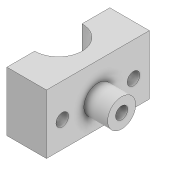
# Autodesk Inventor part: Tube_innerhole_template_p2
Saved by Autodesk Inventor 2022 (Build 260153000, 153)
## iProperties
Created: 2022-05-02
Part Number: Tube_innerhole_template_p2
Material: Generic
Document SubType Name: Modeling
Designer: dell
Density: 1 g/cm^3
Appearance: Default
Author: dell
Autodesk Inventor part; units mm, degrees
ref_plane "YZ Plane" through (0, 0, 0) normal (1, 0, 0) x (0, 1, 0)
ref_plane "XZ Plane" through (0, 0, 0) normal (0, 1, 0) x (-1, 0, 0)
ref_plane "XY Plane" through (0, 0, 0) normal (0, 0, 1) x (1, 0, 0)
sketch "Sketch1" plane through (0, 0, 0) normal (0, 1, 0) x (-1, 0, 0)
  circle A0 centre (0, 0) radius 6
  line L0 (10, 13) -> (-10, 13)
  line L1 (-10, 13) -> (-10, -13)
  line L2 (-10, -13) -> (10, -13)
  line L3 (10, -13) -> (10, 13)
  dimension "d0" = 12
  dimension "d1" = 10
  dimension "d2" = 10
  dimension "d3" = 13
  dimension "d4" = 13
  constraints: 8 end point, 2 parallel, 1 centre point, 1 coincident, 1 horizontal, 1 perpendicular
  measures "d0" diameter of A0
  measures "d1" distance from line of point (0, 0) L1
  measures "d2" distance from line of point (0, 0) L3
  measures "d3" distance from line of point (0, 0) L2
  measures "d4" distance from line of point (0, 0) L0
extrude "Extrusion1" add sketch "Sketch1" along normal blind 15
sketch "Sketch2" plane through (10, 0, 13) normal (1, 0, 0) x (0, 0, -1)
  circle A0 centre (13, 6.5) radius 1.55
  line L0 (0, 0) -> (26, 0) projected
  line L1 (0, 0) -> (0, 15) projected
  point P0 (13, 0)
  dimension "d7" = 3.1
  dimension "d8" = 6.5
  dimension "d11" = 13
  constraints: 1 centre point
  measures "d7" diameter of A0
  measures "d8" distance from line of L0 A0.centre
  measures "d11" distance from line of L1 A0.centre
extrude "Extrusion2" cut sketch "Sketch2" against normal blind 55
sketch "Sketch3" plane through (10, 0, 13) normal (1, 0, 0) x (0, 0, -1)
  circle A0 centre (13, 6.5) radius 1.55 projected
  line L0 (0, 0) -> (26, 0) projected
  line L1 (26, 0) -> (26, 15) projected
  line L2 (0, 15) -> (26, 15) projected
  line L3 (0, 0) -> (0, 15) projected
  circle A1 centre (13, 6.5) radius 3.55
  circle A2 centre (4, 6.5) radius 1.6
  circle A3 centre (22, 6.5) radius 1.6
  point P0 (13, 0)
  dimension "d16" = 2
  dimension "d21" = 3.2
  dimension "d22" = 3.2
  dimension "d23" = 4
  dimension "d24" = 4
  constraints: 3 centre point, 2 horizontal alignment
  measures "d16" radial gap between concentric circles of A0 A1
  measures "d21" diameter of A2
  measures "d22" diameter of A3
  measures "d23" distance from line of L3 A2.centre
  measures "d24" distance from line of L1 A3.centre
extrude "Extrusion3" add sketch "Sketch3" along normal blind 6 contours A1
extrude "Extrusion4" cut sketch "Sketch3" against normal blind 100 contours A2 | A3
sketch "Sketch5" plane through (0, 0, 0) normal (0, -1, 0) x (1, 0, 0)
  line L0 (0, 24.0189) -> (-16.1408, 24.0189)
  line L1 (-16.1408, 24.0189) -> (-16.1408, -21.0721)
  line L2 (-16.1408, -21.0721) -> (0, -21.0721)
  line L3 (0, -21.0721) -> (0, 24.0189)
  line L4 (-34.0392, -28.4766) -> (44.2391, -28.4766)
  line L5 (44.2391, -28.4766) -> (44.2391, 41.3945)
  line L6 (44.2391, 41.3945) -> (-34.0392, 41.3945)
  line L7 (-34.0392, 41.3945) -> (-34.0392, -28.4766)
  point P0 (0, 0)
  constraints: 16 end point, 4 parallel, 2 horizontal, 2 perpendicular
extrude "Extrusion5" cut sketch "Sketch5" against normal blind 100 contours L3 L2 L1 L0
body "Solid1"
